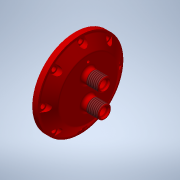
# Autodesk Inventor part: Pump-Motor-CW-Rotation:Case 101
Saved by Autodesk Inventor 2022 (Build 260153000, 153)
## iProperties
Created: 2025-06-16
Document SubType Name: Modeling
Density: 7.25 g/cm^3
Material: Cast Iron
Mass: 939.214 g
Surface Area: 403.338 cm^2
Volume: 129.547 cm^3
Appearance: Red
Designer: cw
Author: cw
Autodesk Inventor part; units mm, degrees
ref_plane "YZ Plane" through (0, 0, 0) normal (1, 0, 0) x (0, 1, 0)
ref_plane "XZ Plane" through (0, 0, 0) normal (0, 1, 0) x (-1, 0, 0)
ref_plane "XY Plane" through (0, 0, 0) normal (0, 0, 1) x (1, 0, 0)
sketch "Sketch1" plane through (0, 0, 0) normal (0, 0, 1) x (1, 0, 0)
  line L0 (0, 0) -> (26.4858, 0)
  line L1 (0, 50) -> (4.6505, 50)
  line L2 (7.9271, 48.2943) -> (11.2766, 43.5107)
  line L3 (12, 41.2164) -> (12, 0)
  line L4 (12, 0) -> (20, 0)
  line L5 (20, 0) -> (20, 43.7388)
  line L6 (8, 64.9614) -> (8, 65)
  line L7 (8, 65) -> (0, 65)
  line L8 (0, 65) -> (0, 50)
  line L9 (8, 65) -> (8, 63.399)
  line L10 (8.7234, 61.1047) -> (19.2766, 46.0331)
  arc A0 (7.9271, 48.2943) -> (4.6505, 50) centre (4.6505, 46) ccw
  arc A1 (12, 41.2164) -> (11.2766, 43.5107) centre (8, 41.2164) ccw
  arc A2 (8, 63.399) -> (8.7234, 61.1047) centre (12, 63.399) ccw
  arc A3 (20, 43.7388) -> (19.2766, 46.0331) centre (16, 43.7388) ccw
  point P0 (20, 45)
  dimension "d0" = 130
  dimension "d1" = 100
  dimension "d2" = 8
  dimension "d4" = 8
  dimension "d5" = 12
  dimension "d7" = 90
  dimension "d10" = 145
  dimension "d11" = 8
  dimension "d12" = 4
  dimension "d13" = 4
  constraints: 22 end point, 8 point on circle, 8 tangent, 5 parallel, 5 point on line, 4 centre point, 3 perpendicular, 2 equal radius, 1 horizontal
  measures "d0" diameter of L7 L0
  measures "d1" diameter of L1.start L0
  measures "d2" distance between parallel lines of L8 L6
  measures "d4" distance between parallel lines of L5 L3
  measures "d5" distance between parallel lines of L8 L3
  measures "d7" diameter of point (20, 45) L0
  measures "d10" angle of L3 L2
  measures "d11" distance between parallel lines of L10 L2
  measures "d12" radius of A0
  measures "d13" radius of A3
revolve "Revolution1" add sketch "Sketch1" angle 360 about axis through (0, 0, 0) along (1, 0, 0)
sketch "Sketch2" plane through (0, 0, 0) normal (-1, 0, 0) x (0, 0, 1)
  circle A0 centre (0, 0) radius 50 projected
  line L0 (0, 0) -> (0, 57) construction
  dimension "d15" = 57
  constraints: 2 end point, 1 coincident, 1 vertical
  measures "d15" distance of L0.start L0.end
hole "Hole1" at (0, 57, 0) direction (1, 0, 0) diameter 7 end through all
sketch "Sketch3" plane through (8, 0, 0) normal (1, 0, 0) x (0, 0, -1)
  circle A0 centre (0, 0) radius 65 projected
  circle A1 centre (0, 57) radius 3.5 projected
  line L0 (-6, 57) -> (-6, 64.7225)
  line L1 (6, 57) -> (6, 64.7225)
  arc A2 (-6, 57) -> (6, 57) centre (0, 57) ccw
  dimension "d89" = 6
  dimension "d90" = 6
  dimension "d91" = 12
  constraints: 4 end point, 4 point on circle, 1 centre point, 1 coincident, 1 parallel, 1 vertical
  measures "d89" radius of A2
  measures "d90" distance from line of A1.centre L0
  measures "d91" distance between parallel lines of L1 L0
extrude "Extrusion1" cut sketch "Sketch3" along normal through all contours L1 A2 L0 A0 picked at (-5.033, 60.1163)
pattern_circular "Circular Pattern1" count 8 over 360 about axis through (4, 0, 0) along (1, 0, 0) of "Hole1", "Extrusion1"
sketch "Sketch4" plane through (20, 0, 0) normal (1, 0, 0) x (0, 0, -1)
  circle A0 centre (0, 0) radius 43.7388 projected
  circle A1 centre (-18, 0) radius 10
  circle A2 centre (18, 0) radius 10
  dimension "d30" = 18
  dimension "d31" = 18
  dimension "d32" = 20
  dimension "d33" = 20
  constraints: 2 centre point, 2 horizontal alignment
  measures "d30" distance of A0.centre A1.centre
  measures "d31" distance of A0.centre A2.centre
  measures "d32" diameter of A1
  measures "d33" diameter of A2
extrude "Extrusion2" add sketch "Sketch4" along normal blind 25 contours A1 | A2
thread "Thread1" size "M20x2.5" class "6g" standard "ANSI Metric M Profile" length 18
thread "Thread2" size "M20x2.5" class "6g" standard "ANSI Metric M Profile" length 18
hole "Hole2" at (45, 0, 18) direction (-1, 0, 0) diameter 8 end through all
hole "Hole3" at (45, 0, -18) direction (-1, 0, 0) diameter 8 end through all
sketch "Sketch6" plane through (0, 0, 0) normal (0, 1, 0) x (-1, 0, 0)
  line L0 (-45, -22) -> (-45, -14) projected
  line L1 (-45, -14) -> (-45, -10)
  line L2 (-45, -10) -> (-42, -10)
  line L3 (-42, -10) -> (-40.5, -11.5)
  line L4 (-40.5, -11.5) -> (-20, -11.5)
  line L5 (-20, -11.5) -> (-20, -18)
  line L6 (-20, -18) -> (-45, -18)
  line L7 (-12, 41.2164) -> (-12, -41.2164) projected
  point P0 (0, 0)
  dimension "d63" = 6.5
  dimension "d64" = 20.5
  dimension "d65" = 8
  dimension "d66" = 135
  dimension "d67" = 8
  dimension "d77" = 3
  constraints: 12 end point, 2 parallel, 1 collinear, 1 midpoint, 1 perpendicular
  measures "d63" distance between parallel lines of L6 L4
  measures "d64" distance of L3.end L4.end
  measures "d65" distance between parallel lines of L7 L5
  measures "d66" angle of L4 L3
  measures "d67" distance between parallel lines of L6 L2
  measures "d77" distance of L1.end L2.end
revolve "Revolution3" cut sketch "Sketch6" angle 360 about axis through (20, 0, -18) along (1, 0, 0)
sketch "Sketch7" plane through (20, 0, 0) normal (1, 0, 0) x (0, 0, -1)
  circle A0 centre (0, 0) radius 43.7388 projected
  point P0 (-36, 0)
  dimension "d69" = 36
  constraints: 1 horizontal alignment
  measures "d69" distance of A0.centre point (-36, 0)
hole "Hole4" at (20, 0, 36) direction (-1, 0, 0) diameter 4 end through all
pattern_linear "Rectangular Pattern1" count 2 spacing 36 along (0, 0, 1) of "Revolution3"
chamfer "Chamfer1" distance 1 angle 45 2 edges at (45, 0, -8) (45, 0, 28)
fillet "Fillet1" radius 4 2 edges at (20, 0, 28) (20, 0, -8)
equation "\"d90\" = d89"
equation "\"d91\" = 2 * d90"
equation "\"d31\" = d30"
body "Solid1"
